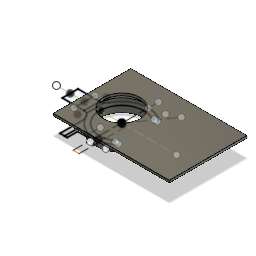
_Op Chamber Slide.1f9aa6c7-411b-427b-a51b-0c5f99999367 (Autodesk Fusion 360 design; units mm, degrees)
Autodesk Fusion 360 part; units mm, degrees
sketch "Sketch1" plane through (0, 0, 0) normal (0, 1, 0) x (1, 0, 0)
  line L0 (-39.5, 0) -> (-39.5, 6)
  line L1 (-39.5, 6) -> (-22.8391, 6)
  line L2 (-50, 0) -> (42, 0) construction
  line L3 (0, 0) -> (18.7964, 26.8441) construction
  arc A0 (9.38, 13.9978) -> (-16.85, 0) centre (0, 0) ccw
  arc A1 (12.8944, 15.7435) -> (-18.3343, 8.8304) centre (0, 0) ccw
  arc A2 (-22.8391, 6) -> (-18.3343, 8.8304) centre (-22.8391, 11) ccw
  line L4 (-28.5277, 8) -> (-28.5277, 0)
  line L5 (-39.5, -6) -> (-22.8391, -6)
  arc A3 (-18.3343, -8.8304) -> (-22.8391, -6) centre (-22.8391, -11) ccw
  line L6 (-28.5277, -8) -> (-28.5277, 0)
  arc A4 (-16.85, 0) -> (9.38, -13.9978) centre (0, 0) ccw
  line L7 (-39.5, 0) -> (-39.5, -6)
  arc A5 (9.8515, 13.8322) -> (12.4661, 13.9912) centre (10.6183, 22.7994) ccw
  line L8 (0, 28) -> (0, 20.2823) construction
  line L9 (0, 20.35) -> (0, -24) construction
  arc A6 (12.4661, 13.9912) -> (12.8944, 15.7435) centre (12.2608, 14.9699) ccw
  arc A7 (9.38, 13.9978) -> (9.8515, 13.8322) centre (9.9367, 14.8285) ccw
  arc A8 (12.8944, -15.7435) -> (12.4661, -13.9912) centre (12.2608, -14.9699) ccw
  arc A9 (12.4661, -13.9912) -> (9.8515, -13.8322) centre (10.6183, -22.7994) ccw
  arc A10 (9.8515, -13.8322) -> (9.38, -13.9978) centre (9.9367, -14.8285) ccw
  line L10 (-0.661, 0) -> (-0.661, -36.4532) construction
  line L11 (3.815, 0) -> (3.815, -36.4532) construction
  line L12 (-0.661, -36.4532) -> (3.815, -36.4532) construction
  line L13 (-0.073, -19.5) -> (-0.073, -20.3)
  line L14 (-0.073, -20.3) -> (3.227, -20.3)
  line L15 (3.227, -19.5) -> (3.227, -20.3)
  arc A11 (3.227, -19.5) -> (-0.073, -19.5) centre (1.577, -19.5) ccw
  line L16 (-0.073, -20.3) -> (-13.423, -20.3)
  line L17 (-13.423, -20.3) -> (-13.423, -30.3)
  line L18 (-13.423, -30.3) -> (-16.923, -30.3)
  line L19 (-5.423, -20.3) -> (-5.423, -11) construction
  arc A12 (-18.3343, -8.8304) -> (-1.4257, -20.3) centre (0, 0) ccw
  arc A13 (1.4257, -20.3) -> (12.8944, -15.7435) centre (0, 0) ccw
  line L20 (-0.073, -22.3) -> (-11.423, -22.3)
  line L21 (-11.423, -22.3) -> (-11.423, -30.3)
  line L22 (-11.423, -30.3) -> (-13.423, -30.3)
  line L23 (-0.073, -22.3) -> (-0.073, -20.3)
  line L24 (-0.073, -20.3) -> (-0.073, -16.8498)
  line L25 (3.227, -20.3) -> (3.227, -16.5381)
  line L26 (-16.923, -30.3) -> (-16.923, -11.302)
  line L27 (-22.8391, -6) -> (-22.8391, 6)
  line L28 (-20.179, -6.7663) -> (-20.179, 6.7663)
  point P0 (-50, 0)
  dimension "d1" = 33.7
  dimension "d4" = 6
  dimension "d5" = 39.5
  dimension "d6" = 3.5
  dimension "d7" = 5
  dimension "d11" = 55
  dimension "d30" = 1
  dimension "d31" = 9
  dimension "d32" = 1
  dimension "d36" = 3.815
  dimension "d37" = 3.3
  dimension "d39" = 0.661
  dimension "d40" = 4.476
  dimension "d41" = 2.238
  dimension "d42" = 0.8
  dimension "d43" = 19.5
  dimension "d44" = 15
  dimension "d45" = 7
  dimension "d46" = 10
  dimension "d47" = 3.5
  dimension "d48" = -2
  dimension "d70" = 28.5277
  constraint coincident L3.start A0.centre
  constraint vertical L0
  constraint perpendicular L0 L1
  constraint horizontal L2
  constraint vertical L8
  constraint coincident L0.start L2
  constraint coincident L2 A0.end
  constraint tangent A1 A2
  constraint tangent L1 A2
  constraint coincident L2 L4.end
  constraint perpendicular L2 L4
  constraint symmetric L3.start L2 A0.centre
  constraint symmetric L0.start L2 L7.start
  constraint symmetric L0.end L2 L5.start
  constraint symmetric P0 L2 L2.start
  constraint symmetric L2 L3.start A0.centre
  constraint symmetric L2 A0.end A4.start
  constraint symmetric L2 A0 A4
  constraint symmetric L2 A1 A12
  constraint symmetric L2 L1.end L5.end
  constraint symmetric L2 A1.end A3.start
  constraint symmetric L2 A2 A3
  constraint symmetric L2 L4.start L6.start
  constraint symmetric L2 L4.end L6.end
  constraint coincident A1 L9.start
  constraint collinear L8 L9
  constraint tangent A1 A6
  constraint tangent A5 A6
  constraint tangent A5 A7
  constraint tangent A0 A7
  constraint equal A6 A7
  constraint symmetric L2 A5 A9
  constraint symmetric L2 A1.start A8.start
  constraint symmetric L2 A5.end A8.end
  constraint symmetric L2 A6 A8
  constraint tangent A9 A10
  constraint tangent A4 A10
  constraint coincident L2 L10.start
  constraint perpendicular L2 L10
  constraint coincident L2 L11.start
  constraint perpendicular L2 L11
  constraint coincident L3.start L9
  constraint perpendicular L11 L12
  constraint tangent L13 A11
  constraint parallel L9 L13
  constraint perpendicular L9 L14
  constraint tangent L15 A11
  constraint perpendicular L14 L15
  constraint perpendicular L13 L16
  constraint perpendicular L16 L17
  constraint perpendicular L17 L18
  constraint coincident L16 L19.start
  constraint perpendicular L16 L19
  constraint coincident L16 A12.end
  constraint concentric A12 A13
  constraint coincident L14 A13.start
  constraint perpendicular L17 L22
  constraint perpendicular L16 L23
  constraint coincident A4 L24.end
  constraint perpendicular L16 L24
  constraint coincident A4 L25.end
  constraint perpendicular L14 L25
  constraint coincident A12 L26.end
  constraint perpendicular L18 L26
  constraint midpoint A3 L28.start
  constraint midpoint A2 L28.end
  measures "d1" diameter of A0
  measures "d4" distance of L0.start L0.end
  measures "d5" distance of L3.start L0
  measures "d6" distance of A0 A1
  measures "d7" radius of A2
  measures "d11" angle of L2 L3
  measures "d30" radius of A6
  measures "d31" radius of A5
  measures "d32" radius of A10
  measures "d36" distance of L9 L11
  measures "d37" diameter of A11
  measures "d39" distance of L9 L10
  measures "d40" distance of L10.end L11.end
  measures "d41" distance of L10 A11.centre
  measures "d42" distance of A11.centre L14 L3.start
  measures "d43" vertical distance of L3.start A11.centre
  measures "d44" distance of A11.centre L17
  measures "d45" distance of A11.centre L19
  measures "d46" distance of L16 L18
  measures "d47" distance of L17.end L18.end
  measures "d70" distance of L4 L3.start
  measures "d118" distance of L3.start
extrude "Extrude1" add sketch "Sketch1" along normal mid plane 10 contours A2 A3 L27 L28 | A0 A1 A2 A3 A4 A5 A6 A7 L13 L16 A12 L24 L28 | L13 L14 L15 A11 A13 L24 L25 | A4 A11 L24 L25 | A4 A8 A9 A10 L15 A13 L25
ref_plane "WorkPlane1" through (-16.85, 0, 0) normal (1, 0, 0) x (0, 1, 0)
sketch "Sketch2" plane through (-16.85, 0, 0) normal (1, 0, 0) x (0, 0, -1)
  line L0 (-1.6743, 2.9) -> (-3.3486, 0)
  line L1 (-3.3486, 0) -> (-1.6743, -2.9)
  line L2 (-1.6743, -2.9) -> (1.6743, -2.9)
  line L3 (1.6743, -2.9) -> (3.3486, 0)
  line L4 (3.3486, 0) -> (1.6743, 2.9)
  line L5 (1.6743, 2.9) -> (-1.6743, 2.9)
  circle A0 centre (0, 0) radius 1.6
  line L6 (-1.175, 2.175) -> (1.175, 2.175)
  line L7 (2.175, 1.175) -> (2.175, -1.175)
  line L8 (1.175, -2.175) -> (-1.175, -2.175)
  line L9 (-2.175, -1.175) -> (-2.175, 1.175)
  line L10 (-2.175, 2.175) -> (2.175, -2.175) construction
  line L11 (2.175, 2.175) -> (-2.175, -2.175) construction
  arc A1 (-1.175, 2.175) -> (-2.175, 1.175) centre (-1.175, 1.175) ccw
  arc A2 (-2.175, -1.175) -> (-1.175, -2.175) centre (-1.175, -1.175) ccw
  arc A3 (1.175, -2.175) -> (2.175, -1.175) centre (1.175, -1.175) ccw
  arc A4 (2.175, 1.175) -> (1.175, 2.175) centre (1.175, 1.175) ccw
  circle A5 centre (0, 2.175) radius 2.25
  dimension "d16" = 2.9
  dimension "d104" = 4.35
  dimension "d105" = 4.35
  dimension "d106" = 1
  dimension "d125" = 4.5
  constraint coincident A0.centre origin
  constraint horizontal L6
  constraint perpendicular L6 L7
  constraint parallel L6 L8
  constraint parallel L7 L9
  constraint coincident L10 A0.centre
  constraint coincident L11 A0.centre
  constraint coincident L10.start L6
  constraint coincident L10.start L9
  constraint tangent L6 A1
  constraint tangent L9 A1
  constraint coincident L11.end L8
  constraint coincident L11.end L9
  constraint tangent L8 A2
  constraint tangent L9 A2
  constraint equal A1 A2
  constraint coincident L10.end L8
  constraint coincident L10.end L7
  constraint tangent L8 A3
  constraint tangent L7 A3
  constraint equal A1 A3
  constraint coincident L11.start L7
  constraint coincident L11.start L6
  constraint tangent L7 A4
  constraint tangent L6 A4
  constraint equal A1 A4
  constraint midpoint L6 A5.centre
  measures "d16" distance of A0.centre L5
  measures "d104" distance of L10.end L11.end
  measures "d105" distance of L11.start L10.end
  measures "d106" radius of A1
  measures "d125" diameter of A5
ref_plane "WorkPlane2" through (0, 4.9, 0) normal (0, 1, 0) x (0, 0, 1)
extrude "Extrude19" add sketch "Sketch1" along normal blind 8.3 contours A2 A3 L27 L28
sketch "Sketch11" plane through (0, 8.3, 0) normal (0, 1, 0) x (-1, 0, 0)
  arc A0 (20.179, 6.7663) -> (22.8391, 6) centre (22.8391, 11) ccw
  line L0 (20.179, 6.7663) -> (20.179, -6.7663)
  arc A1 (22.8391, -6) -> (20.179, -6.7663) centre (22.8391, -11) ccw
  line L1 (22.8391, -6) -> (22.8391, 6)
  line L2 (22.8391, -29.79) -> (-66.1609, -29.79)
  line L3 (-66.1609, -29.79) -> (-66.1609, 29.79)
  line L4 (-66.1609, 29.79) -> (22.8391, 29.79)
  line L5 (22.8391, 29.79) -> (22.8391, -29.79)
  line L6 (22.8391, 6) -> (22.8391, -6)
  point P0 (22.8391, -6)
  dimension "d116" = 89
  dimension "d117" = 59.58
  dimension "d118" = 29.79
  constraint horizontal L2
  constraint vertical L3
  constraint horizontal L4
  constraint vertical L5
  constraint coincident L5 P0
  measures "d116" distance of L2.start L2.end
  measures "d117" distance of L2.end L3.end
  measures "d118" distance of origin L2
extrude "Extrude20" add sketch "Sketch11" along normal blind 1.83
sketch "Sketch12" plane through (0, -5, 0) normal (0, -1, 0) x (1, 0, 0)
  arc A0 (-1.4257, 20.3) -> (-18.3343, 8.8304) centre (0, 0) ccw
  arc A1 (-22.8391, 6) -> (-18.3343, 8.8304) centre (-22.8391, 11) ccw
  line L0 (-22.8391, 6) -> (-22.8391, -6)
  arc A2 (-18.3343, -8.8304) -> (-22.8391, -6) centre (-22.8391, -11) ccw
  arc A3 (-18.3343, -8.8304) -> (12.8944, -15.7435) centre (0, 0) ccw
  arc A4 (12.8944, -15.7435) -> (12.4661, -13.9912) centre (12.2608, -14.9699) ccw
  arc A5 (12.4661, -13.9912) -> (9.8515, -13.8322) centre (10.6183, -22.7994) ccw
  arc A6 (9.8515, -13.8322) -> (9.38, -13.9978) centre (9.9367, -14.8285) ccw
  arc A7 (9.38, 13.9978) -> (9.38, -13.9978) centre (0, 0) ccw
  arc A8 (9.38, 13.9978) -> (9.8515, 13.8322) centre (9.9367, 14.8285) ccw
  arc A9 (9.8515, 13.8322) -> (12.4661, 13.9912) centre (10.6183, 22.7994) ccw
  arc A10 (12.4661, 13.9912) -> (12.8944, 15.7435) centre (12.2608, 14.9699) ccw
  arc A11 (12.8944, 15.7435) -> (1.4257, 20.3) centre (0, 0) ccw
  line L1 (1.4257, 20.3) -> (-1.4257, 20.3)
  arc A12 (-16.85, 0) -> (9.38, -13.9978) centre (0, 0) ccw
  arc A13 (9.38, 13.9978) -> (-16.85, 0) centre (0, 0) ccw
  circle A14 centre (0, 0) radius 14
  dimension "d128" = 28
  constraint concentric A0 A14
  measures "d128" diameter of A14
extrude "Extrude22" cut sketch "Sketch12" against normal up to surface (15.13 mm away) contours A14
equation "d5 = 50 mm - 10.5 mm"
equation "d41 = ( 4.476 / 2 ) * 1 mm"
equation "d43 = d1 / 2 + 1 mm + d37 / 2"
equation "d114 = 7.4 mm + 0.9 mm"
equation "d118 = d117 / 2"
equation "d120 = 2.23 mm - 0.4 mm"
equation "d119 = ( 30 / 2 ) * 1 mm + 7 mm"
equation "d95 = 0.5 mm + 0.8 mm"
